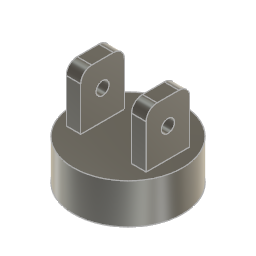
screw holder v10 (Autodesk Fusion 360 design; units mm, degrees)
Autodesk Fusion 360 part; units mm, degrees
sketch "Sketch1" plane through (0, 0, 0) normal (0, 0, 1) x (1, 0, 0)
  circle A0 centre (0, 0) radius 15
  dimension "d1" = 30
  constraint coincident A0.centre origin
  measures "d1" diameter of A0
extrude "Extrude1" add sketch "Sketch1" along normal blind 11
sketch "Sketch2" plane through (0, 0, 11) normal (0, 0, 1) x (-1, 0, 0)
  circle A0 centre (0, 0) radius 15
  circle A1 centre (0, 0) radius 3
  dimension "d5" = 6
  constraint coincident A0.centre A1.centre
  measures "d5" diameter of A1
extrude "Extrude2" cut sketch "Sketch2" against normal blind 8 contours A1
ref_plane "WorkPlane3" through (0, 11, 0) normal (0, 1, 0) x (0, 0, 1)
ref_plane "WorkPlane4" through (0, -11, 0) normal (0, 1, 0) x (0, 0, 1)
move_body "Move1" bodies 1 to x (-1, 0, 0) y (0, 1, 0) z (0, 0, -1) at (0, 0, 22)
sketch "Sketch13" plane through (0, 0, 22) normal (0, 0, 1) x (-1, 0, 0)
  circle A0 centre (0, 0) radius 15
  line L0 (11, -6) -> (11, 6)
  line L1 (-11, -6) -> (-11, 6)
  line L2 (-11, -6) -> (-7, -6)
  line L3 (-7, -6) -> (-7, 6)
  line L4 (-7, 6) -> (-11, 6)
  line L5 (11, -6) -> (7, -6)
  line L6 (7, -6) -> (7, 6)
  line L7 (7, 6) -> (11, 6)
  point P0 (15, 0)
  point P1 (-15, 0)
  point P2 (-0.0376, -15)
  dimension "d60" = 12
  dimension "d61" = 4
  dimension "d64" = 4
  dimension "d65" = 4
  dimension "d66" = 4
  dimension "d68" = 9
  dimension "d69" = 9
  constraint coincident A0 P0
  constraint vertical L0
  constraint vertical L1
  constraint coincident A0 P1
  constraint perpendicular L1 L2
  constraint perpendicular L2 L3
  constraint perpendicular L1 L4
  constraint perpendicular L0 L5
  constraint perpendicular L5 L6
  constraint coincident A0 P2
  measures "d60" distance of L0.start L0.end
  measures "d61" distance of P0 L0
  measures "d64" distance of L1 P1
  measures "d65" distance of L1.start L2.end
  measures "d66" distance of L0.start L5.end
  measures "d68" distance of L5 P2
  measures "d69" distance of L2 P2
extrude "Extrude12" add sketch "Sketch13" along normal blind 15 contours L0 L5 L6 L7 | L1 L2 L3 L4
sketch "Sketch14" plane through (11, 0, 0) normal (1, 0, 0) x (0, 1, 0)
  line L0 (-6, 22) -> (6, 22)
  line L1 (6, 22) -> (6, 37)
  line L2 (6, 37) -> (-6, 37)
  line L3 (-6, 37) -> (-6, 22)
  circle A0 centre (0, 30) radius 1.8
  dimension "d72" = 3.6
  dimension "d73" = 7
  measures "d72" diameter of A0
  measures "d73" distance of L2 A0.centre
extrude "Extrude13" cut sketch "Sketch14" against normal blind 28 contours A0
fillet "Fillet1" radius 3 1 edges at (9, -6, 37)
fillet "Fillet2" radius 3 1 edges at (9, 6, 37)
fillet "Fillet3" radius 3 2 edges at (-9, 6, 37) (-9, -6, 37)
